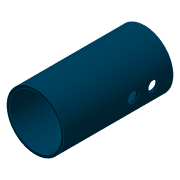
# Autodesk Inventor part: 8,5 hub
Saved by Autodesk Inventor 2018 (Build 220112000, 112)
## iProperties
Created: 2019-12-18
Part Number: 8,5 hub
Material: Generic
Document SubType Name: Modeling
Designer: Ibnu
Density: 1 g/cm^3
Appearance: Default
Author: Ibnu
Autodesk Inventor part; units mm, degrees
ref_plane "XZ Plane" through (0, 0, 0) normal (0, 1, 0) x (-1, 0, 0)
ref_plane "XY Plane" through (0, 0, 0) normal (0, 0, 1) x (1, 0, 0)
sketch "Sketch1" plane through (0, 0, 0) normal (0, 1, 0) x (-1, 0, 0)
  circle A0 centre (0, 0) radius 13
  circle A1 centre (0, 0) radius 14.35
  dimension "d0" = 26
  dimension "d2" = 28.7
  constraints: 2 centre point
  measures "d0" diameter of A0
  measures "d2" diameter of A1
extrude "Extrusion1" add sketch "Sketch1" along normal blind 55
ref_plane "Work Plane1" through (14.35, 0, 0) normal (1, 0, 0) x (0, 1, 0)
sketch "Sketch2" plane through (14.35, 0, 0) normal (1, 0, 0) x (0, 1, 0)
  circle A0 centre (35, 0) radius 2.5
  circle A1 centre (45, 0) radius 2.5
  point P0 (0, 0)
  constraints: 2 centre point
extrude "Extrusion2" cut sketch "Sketch2" against normal through all
body "Solid1"
